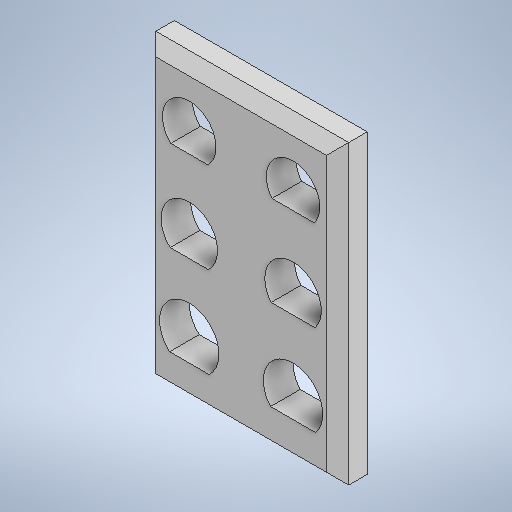
# Autodesk Inventor part: N20shaft_sizing
Saved by Autodesk Inventor 2025.2 (Build 292293000, 293)
## iProperties
Created: 2025-03-05
Part Number: N20shaft_sizing
Material: Generic
Document SubType Name: Modeling
Designer: 3lin2
Density: 1 g/cm^3
Appearance: Default
Author: 3lin2
Autodesk Inventor part; units mm, degrees
ref_plane "YZ Plane" through (0, 0, 0) normal (1, 0, 0) x (0, 1, 0)
ref_plane "XZ Plane" through (0, 0, 0) normal (0, 1, 0) x (-1, 0, 0)
ref_plane "XY Plane" through (0, 0, 0) normal (0, 0, 1) x (1, 0, 0)
sketch "Sketch1" plane through (0, 0, 0) normal (0, 0, 1) x (1, 0, 0)
  line L0 (-9.9986, 9.999) -> (3.0014, 9.999)
  line L1 (3.0014, 9.999) -> (3.0014, -10.001)
  line L2 (3.0014, -10.001) -> (-9.9986, -10.001)
  line L3 (-9.9986, -10.001) -> (-9.9986, 9.999)
  point P0 (0.0014, -0.001)
  point P1 (0.0014, -0.001)
  point P2 (-9.9986, -0.001)
  dimension "d0" = 13
  dimension "d1" = 20
  dimension "d2" = 10
  dimension "d3" = 10
  constraints: 8 end point, 2 parallel, 1 coincident, 1 horizontal, 1 midpoint, 1 perpendicular
  measures "d0" distance between parallel lines of L1 L3
  measures "d1" distance between parallel lines of L2 L0
  measures "d2" distance of point (-9.999, -0.001) point (0.001, -0.001)
  measures "d3" distance from line of point (0.001, -0.001) L0
extrude "Extrusion1" add sketch "Sketch1" along normal blind 2
sketch "Sketch4" plane through (0, 0, 2) normal (0, 0, 1) x (1, 0, 0)
  line L0 (3.0014, 9.999) -> (-9.9986, 9.999) projected
  line L1 (-9.9986, 9.999) -> (-9.9986, -10.001) projected
  point P0 (-6.9986, 5.999)
  point P1 (0.0014, 5.999)
  dimension "d20" = 4
  dimension "d21" = 3
  dimension "d29" = 4
  measures "d20" distance from line of point (-6.999, 5.999) L0
  measures "d21" distance from line of L1 point (-6.999, 5.999)
  measures "d29" distance from line of L0 point (0.001, 5.999)
hole "Hole3" at (-6.9986, 5.999, 2) at (0.0014, 5.999, 2) direction (0, 0, -1) diameter 3.6 end through all
sketch "Sketch7" plane through (0, 0, 2) normal (0, 0, 1) x (1, 0, 0)
  circle A0 centre (-6.9986, 5.999) radius 1.8 projected
  line L0 (-8.2436, 4.699) -> (-5.7536, 4.699)
  point P0 (0, 0)
  point P1 (-6.9986, 4.699)
  constraints: 2 end point, 2 point on circle, 1 horizontal, 1 midpoint
extrude "Extrusion2" add sketch "Sketch7" against normal blind 2 contours L0 A0 picked at (-7.3099, 4.6194)
sketch "Sketch8" plane through (0, 0, 2) normal (0, 0, 1) x (1, 0, 0)
  circle A0 centre (0.0014, 5.999) radius 1.8 projected
  line L0 (-1.4234, 4.899) -> (1.4262, 4.899)
  point P0 (0, 0)
  point P1 (0.0014, 4.899)
  dimension "d58" = 1.1
  constraints: 2 end point, 2 point on circle, 1 horizontal, 1 midpoint
  measures "d58" distance of point (0.001, 4.899) A0.centre
extrude "Extrusion3" add sketch "Sketch8" against normal blind 2 contours L0 A0 picked at (0.381, 4.801)
sketch "Sketch5" plane through (0, 0, 2) normal (0, 0, 1) x (1, 0, 0)
  line L0 (-9.9986, 9.999) -> (-9.9986, -10.001) projected
  point P0 (0, 0)
  point P1 (-6.9986, 0)
  point P2 (0, 0)
  point P3 (-9.9986, -0.001)
  dimension "d37" = 3
  constraints: 1 coincident, 1 midpoint
  measures "d37" distance of point (-9.999, -0.001) point (-6.999, 0)
hole "Hole4" at (-6.9986, 0, 2) at (0, 0, 2) direction (0, 0, -1) diameter 3.8 end through all
sketch "Sketch9" plane through (0, 0, 2) normal (0, 0, 1) x (1, 0, 0)
  circle A0 centre (-6.9986, 0) radius 1.9 projected
  line L0 (-8.2831, -1.4) -> (-5.7141, -1.4)
  circle A1 centre (0, 0) radius 1.9 projected
  line L1 (-1.4731, -1.2) -> (1.4731, -1.2)
  point P0 (-6.9986, -1.4)
  point P1 (0, -1.2)
  dimension "d61" = 1.4
  dimension "d62" = 1.2
  constraints: 4 end point, 4 point on circle, 2 horizontal, 2 midpoint
  measures "d61" distance of point (-6.999, -1.4) A0.centre
  measures "d62" distance of point (0, -1.2) point (0, 0)
extrude "Extrusion4" add sketch "Sketch9" against normal blind 2 contours L0 A0 | L1 A1 picked at (-7.2994, -1.4907) picked at (0.391, -1.2982)
sketch "Sketch6" plane through (0, 0, 2) normal (0, 0, 1) x (1, 0, 0)
  line L0 (-9.9986, 9.999) -> (-9.9986, -10.001) projected
  line L1 (-9.9986, -10.001) -> (3.0014, -10.001) projected
  point P0 (0, 0)
  point P1 (-6.9986, -6.001)
  point P2 (0, -6.001)
  dimension "d45" = 3
  dimension "d46" = 4
  dimension "d47" = 4
  measures "d45" distance from line of L0 point (-6.999, -6.001)
  measures "d46" distance from line of L1 point (-6.999, -6.001)
  measures "d47" distance from line of L1 point (0, -6.001)
hole "Hole5" at (-6.9986, -6.001, 2) at (0, -6.001, 2) direction (0, 0, -1) diameter 4 end through all
sketch "Sketch10" plane through (0, 0, 2) normal (0, 0, 1) x (1, 0, 0)
  circle A0 centre (-6.9986, -6.001) radius 2 projected
  line L0 (-8.3215, -7.501) -> (-5.6757, -7.501)
  circle A1 centre (0, -6.001) radius 2 projected
  line L1 (-1.5199, -7.301) -> (1.5199, -7.301)
  point P0 (0, 0)
  point P1 (-6.9986, -7.501)
  point P2 (0, -7.301)
  dimension "d65" = 1.5
  dimension "d66" = 1.3
  constraints: 4 end point, 4 point on circle, 2 horizontal, 2 midpoint
  measures "d65" distance of point (-6.999, -7.501) A0.centre
  measures "d66" distance of point (0, -7.301) A1.centre
extrude "Extrusion5" add sketch "Sketch10" against normal blind 2 contours L0 A0 | L1 A1 picked at (-7.3075, -7.5918) picked at (-0.3855, -7.4116)
chamfer "Chamfer1" distance 0.75 angle 45 4 edges at (-3.4986, 9.999, 2) (-3.4986, -10.001, 2) (3.0014, -0.001, 2) (-9.9986, -0.001, 2)
body "Solid1"
